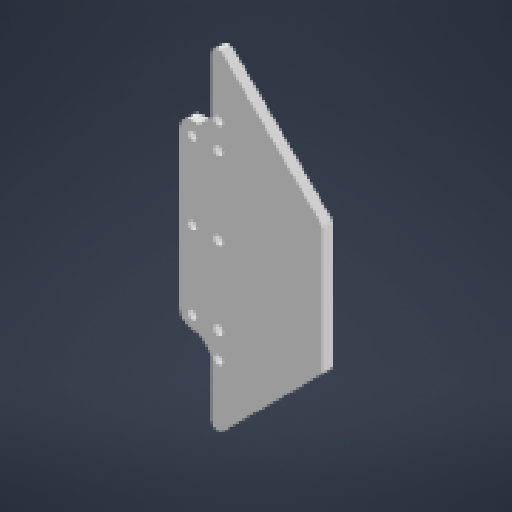
# Autodesk Inventor part: wedge
Saved by Autodesk Inventor 2025.2 (Build 292293000, 293)
## iProperties
Created: 2025-12-02
Part Number: wedge
Material: Generic
Document SubType Name: Modeling
Designer: cloudy
Density: 1 g/cm^3
Appearance: Default
Author: cloudy
Autodesk Inventor part; units mm, degrees
ref_plane "YZ Plane" through (0, 0, 0) normal (1, 0, 0) x (0, 1, 0)
ref_plane "XZ Plane" through (0, 0, 0) normal (0, 1, 0) x (-1, 0, 0)
ref_plane "XY Plane" through (0, 0, 0) normal (0, 0, 1) x (1, 0, 0)
sketch "Sketch1" plane through (0, 0, 0) normal (0, 0, 1) x (1, 0, 0)
  line L0 (88.9, 0) -> (-12.7, 101.6)
  line L1 (-12.7, 101.6) -> (-12.7, -101.6)
  line L2 (-12.7, -101.6) -> (88.9, 0)
  line L3 (-12.7, 0) -> (88.9, 0)
  line L4 (57.4343, 183.898) -> (-323.5657, 183.898)
  line L5 (-323.5657, 183.898) -> (-323.5657, -183.898)
  line L6 (-323.5657, -183.898) -> (57.4343, -183.898)
  line L7 (57.4343, -183.898) -> (57.4343, 183.898)
  line L8 (57.4343, 183.898) -> (-323.5657, -183.898) construction
  line L9 (-323.5657, 183.898) -> (57.4343, -183.898) construction
  circle A0 centre (6.35, 38.1) radius 2.1844 projected
  circle A1 centre (-6.35, 38.1) radius 2.1844 projected
  circle A2 centre (-6.35, -38.1) radius 2.1844 projected
  circle A3 centre (6.35, -38.1) radius 2.1844 projected
  circle A4 centre (6.35, 0) radius 2.1844 projected
  circle A5 centre (6.35, 88.9) radius 2.1844 projected
  circle A6 centre (6.35, 50.8) radius 2.1844 projected
  circle A7 centre (6.35, -50.8) radius 2.1844 projected
  circle A8 centre (-6.35, 0) radius 2.1844 projected
  circle A9 centre (-6.35, 38.1) radius 6.35
  circle A10 centre (-6.35, -38.1) radius 6.35
  line L10 (3.175, -85.725) -> (3.175, -44.45)
  line L11 (3.175, -44.45) -> (-11.204, -44.45)
  line L12 (-10.742, 44.45) -> (3.175, 44.45)
  line L13 (3.175, 44.45) -> (3.175, 85.725)
  point P0 (0, 0)
  point P1 (-133.0657, 0)
  point P2 (57.4343, 31.4657)
  point P3 (-6.35, 44.45)
  point P4 (-12.7, 38.1)
  point P5 (-12.7, -38.1)
  point P6 (-6.35, -44.45)
  point P7 (57.4343, -31.4657)
  dimension "d0" = 101.6
  dimension "d2" = 381
  dimension "d4" = 12.7
  dimension "d5" = 12.7
  dimension "d6" = 3.175
  dimension "d7" = 3.175
  constraints: 28 end point, 4 vertical, 3 horizontal, 3 midpoint, 3 perpendicular, 3 point on line, 3 tangent, 2 centre point, 2 coincident, 2 parallel
  measures "d0" distance of L3.start L0.start
  measures "d2" distance of L5.end L6.end
  measures "d4" diameter of A9
  measures "d5" diameter of A10
  measures "d6" distance from line of A7.centre L10
  measures "d7" distance from line of L13 A6.centre
extrude "Extrusion1" add sketch "Sketch1" along normal blind 5.08 contours L0 L7 L3 A4 A8 L1 A9 L12 L13 | A9 | L7 L2 L10 L11 A10 L1 L3 A8 A4 | A10
chamfer "Chamfer1" distance 6.35 angle 45 2 edges at (3.175, 44.45, 2.54) (3.175, -44.45, 2.54)
fillet "Fillet1" radius 3.175 4 edges at (3.175, 85.725, 2.54) (3.175, -85.725, 2.54) (57.4343, 31.4657, 2.54) (57.4343, -31.4657, 2.54)
body "Solid1"
